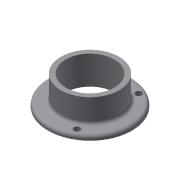
# Autodesk Inventor part: 00_Zeiss_eyepieceport
Saved by Autodesk Inventor 2019.4 (Build 234330000, 330)
## iProperties
Created: 2020-07-06
Part Number: 00_Zeiss_eyepieceport
Material: Generic
Document SubType Name: Modeling
Designer: diederichbenedict
Density: 1 g/cm^3
Appearance: Default
Author: diederichbenedict
Autodesk Inventor part; units mm, degrees
ref_plane "YZ Plane" through (0, 0, 0) normal (1, 0, 0) x (0, 1, 0)
ref_plane "XZ Plane" through (0, 0, 0) normal (0, 1, 0) x (-1, 0, 0)
ref_plane "XY Plane" through (0, 0, 0) normal (0, 0, 1) x (1, 0, 0)
sketch "Sketch1" plane through (0, 0, 0) normal (0, 1, 0) x (-1, 0, 0)
  circle A0 centre (0, 0) radius 26.45
  circle A1 centre (22.45, 0) radius 2
  circle A2 centre (0, 0) radius 22.45 construction
  circle A3 centre (-11.225, 19.4423) radius 2
  circle A4 centre (-11.225, -19.4423) radius 2
  circle A5 centre (0, 0) radius 15.35
  dimension "d0" = 52.9
  dimension "d1" = 4
  dimension "d2" = 4
  dimension "d5" = 360
  dimension "d7" = 30.7
  constraints: 5 centre point, 3 coincident, 1 horizontal alignment, 9 other
  measures "d0" diameter of A0
  measures "d1" diameter of A1
  measures "d7" diameter of A5
extrude "Extrusion1" add sketch "Sketch1" along normal blind 3
sketch "Sketch2" plane through (0, 3, 0) normal (0, 1, 0) x (1, 0, 0)
  circle A0 centre (0, 0) radius 15.35 projected
  circle A1 centre (11.225, 19.4423) radius 2 projected
  circle A2 centre (11.225, -19.4423) radius 2 projected
  circle A3 centre (-22.45, 0) radius 2 projected
  circle A4 centre (0, 0) radius 26.45 projected
  circle A5 centre (0, 0) radius 18.35
  dimension "d10" = 3
  constraints: 1 centre point
  measures "d10" radial gap between concentric circles of A0 A5
extrude "Extrusion2" add sketch "Sketch2" along normal blind 15 contours A5
fillet "Fillet1" radius 2 2 edges at (-18.35, 3, 0) (26.45, 3, 0)
body "Solid1"
